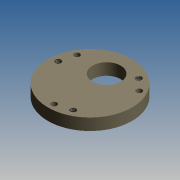
# Autodesk Inventor part: P21
Saved by Autodesk Inventor 2012 SP1 (Build 160190100, 190)
## iProperties
Created: 2012-07-09
Part Number: P21
Material: Aluminium
Document SubType Name: Modeling
Designer: sta
Density: 2.7 g/cm^3
Description: Adaptateur_Moteur
Mass: 11.5794 g
Surface Area: 27.9343 cm^2
Volume: 4.28867 cm^3
Author: sta
Title: Kart 2012
Autodesk Inventor part; units mm, degrees
ref_plane "YZ Plane" through (0, 0, 0) normal (1, 0, 0) x (0, 1, 0)
ref_plane "XZ Plane" through (0, 0, 0) normal (0, 1, 0) x (-1, 0, 0)
ref_plane "XY Plane" through (0, 0, 0) normal (0, 0, 1) x (1, 0, 0)
sketch "Sketch1" plane through (0, 0, 0) normal (0, 0, 1) x (1, 0, 0)
  circle A0 centre (0, 0) radius 18
  circle A1 centre (0, 7.12) radius 6
  line L0 (0, 0) -> (0, 7.12) construction
  dimension "d0" = 36
  dimension "d1" = 12
  dimension "d2" = 7.12
  constraints: 2 centre point, 2 end point, 1 coincident, 1 vertical
  measures "d0" diameter of A0
  measures "d1" diameter of A1
  measures "d2" distance of L0.start L0.end
extrude "Extrusion1" add sketch "Sketch1" along normal mid plane 5
sketch "Sketch2" plane through (0, 0, -2.5) normal (0, 0, -1) x (-1, 0, 0)
  circle A0 centre (0, 0) radius 15.425 construction
  circle A1 centre (0, 7.12) radius 6 construction
  line L0 (0, 7.12) -> (0, 7.7125) construction
  point P0 (0, -15.425)
  point P1 (13.3584, 7.7125)
  point P2 (-13.3584, 7.7125)
  dimension "d11" = 360
  constraints: 2 end point, 1 centre point, 1 coincident, 4 other
hole "Hole1" at (0, -15.425, -2.5) at (-13.3584, 7.7125, -2.5) at (13.3584, 7.7125, -2.5) direction (0, 0, 1) diameter 2.4 end through all counterbore diameter 4.4 counterbore depth 3
sketch "Sketch3" plane through (0, 0, -2.5) normal (0, 0, -1) x (-1, 0, 0)
  circle A0 centre (-13.3584, 7.7125) radius 2.2 construction
  circle A1 centre (-13.3584, 7.7125) radius 1.2 construction
  line L0 (-13.3584, 7.7125) -> (0, 0) construction
  line L1 (0, 0) -> (-9.6467, 13.7769) construction
  circle A2 centre (0, 0) radius 15.425 construction
  circle A3 centre (0, 7.12) radius 6 construction
  line L2 (0, 0) -> (0, 7.12) construction
  point P0 (-8.6036, 12.2873)
  dimension "d37" = 30.85
  dimension "d20" = 25
  dimension "d21" = 15
  dimension "d38" = 60
  dimension "d39" = 7.12
  constraints: 6 end point, 1 coincident, 1 point on line, 1 vertical, 3 other
  measures "d20" angle of L0 L1
  measures "d21" distance of L0.end point (-8.604, 12.287)
  measures "d38" angle of L0 L2
  measures "d39" distance of L2.end L0.end
hole "Hole2" at (8.6036, 12.2873, -2.5) direction (0, 0, 1) diameter 2.459 end through all thread size "M3x0.5" class "6H" standard "ISO Metric profile"
pattern_circular "Circular Pattern1" count 3 over 360 about axis through (0, 0, 0) along (0, 0, 1) of "Hole2"
body "Solid1"
